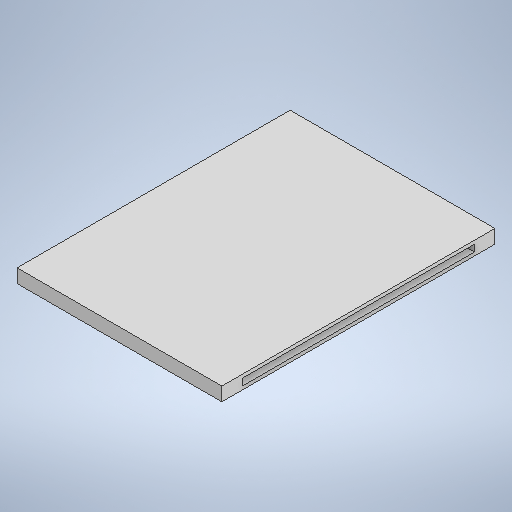
# Autodesk Inventor part: Chassis Upper - Female
Saved by Autodesk Inventor 2025.2 (Build 292293000, 293)
## iProperties
Created: 2025-01-18
Part Number: Chassis Upper - Female
Material: Generic
Document SubType Name: Modeling
Designer: mtidd
Density: 1 g/cm^3
Appearance: Default
Author: mtidd
Autodesk Inventor part; units mm, degrees
ref_plane "YZ Plane" through (0, 0, 0) normal (1, 0, 0) x (0, 1, 0)
ref_plane "XZ Plane" through (0, 0, 0) normal (0, 1, 0) x (-1, 0, 0)
ref_plane "XY Plane" through (0, 0, 0) normal (0, 0, 1) x (1, 0, 0)
sketch "Sketch1" plane through (0, 0, 0) normal (0, 1, 0) x (-1, 0, 0)
  line L0 (0, 0) -> (150, 0)
  line L1 (150, 0) -> (150, -200)
  line L2 (150, -200) -> (0, -200)
  line L3 (0, -200) -> (0, 0)
  dimension "d0" = 150
  dimension "d1" = 200
  constraints: 8 end point, 2 parallel, 1 horizontal, 1 perpendicular
  measures "d0" distance of L1.end L2.end
  measures "d1" distance of L0.end L1.end
extrude "Extrusion1" add sketch "Sketch1" along normal blind 10
sketch "Sketch2" plane through (0, 0, 0) normal (1, 0, 0) x (0, 0, -1)
  line L0 (15, 2.5) -> (185, 2.5)
  line L1 (185, 2.5) -> (185, 7.5)
  line L2 (185, 7.5) -> (15, 7.5)
  line L3 (15, 7.5) -> (15, 2.5)
  point P0 (0, 0)
  dimension "d4" = 170
  dimension "d5" = 5
  constraints: 8 end point, 2 parallel, 1 horizontal, 1 perpendicular
  measures "d4" distance of L2.end L1.end
  measures "d5" distance of L1.end L0.end
extrude "Extrusion2" cut sketch "Sketch2" against normal blind 25
body "Solid1"
